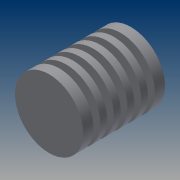
# Autodesk Inventor part: Ceramic_Spacer
Saved by Autodesk Inventor 2015 SP1 (Build 190203100, 203)
## iProperties
Created: 2015-09-10
Part Number: Ceramic_Spacer
Material: Generic
Document SubType Name: Modeling
Designer: nfitch
Density: 1 g/cm^3
Appearance: Default
Author: nfitch
Autodesk Inventor part; units mm, degrees
ref_plane "YZ Plane" through (0, 0, 0) normal (1, 0, 0) x (0, 1, 0)
ref_plane "XZ Plane" through (0, 0, 0) normal (0, 1, 0) x (-1, 0, 0)
ref_plane "XY Plane" through (0, 0, 0) normal (0, 0, 1) x (1, 0, 0)
sketch "Sketch1" plane through (0, 0, 0) normal (0, 1, 0) x (-1, 0, 0)
  circle A0 centre (0, 0) radius 5
  dimension "d0" = 10
  constraints: 1 centre point, 1 coincident
  measures "d0" diameter of A0
extrude "Extrusion1" add sketch "Sketch1" along normal blind 12
sketch "Sketch2" plane through (0, 0, 0) normal (1, 0, 0) x (0, 1, 0)
  line L0 (1.5, -2.5) -> (2.5, -2.5)
  line L1 (2.5, -2.5) -> (2.5, -7.5)
  line L2 (2.5, -7.5) -> (1.5, -7.5)
  line L3 (1.5, -7.5) -> (1.5, -2.5)
  line L4 (0, -5) -> (12, -5) projected
  line L5 (1.5, -2.5) -> (2.5, -7.5) construction
  line L6 (2.5, -2.5) -> (1.5, -7.5) construction
  line L7 (0, 0) -> (12, 0)
  line L8 (12, -5) -> (12, 5) projected
  line L9 (0, -10) -> (0, 7.5) projected
  line L10 (-2.4, 0) -> (14.4, 0) projected
  point P0 (2, -5)
  dimension "d3" = 1
  dimension "d4" = 5
  dimension "d9" = 2
  constraints: 14 end point, 3 midpoint, 2 parallel, 1 horizontal, 1 perpendicular, 1 point on line
  measures "d3" distance of L1.end L2.end
  measures "d4" distance of L0.end L1.end
  measures "d9" distance from line of L9 point (2, -5)
revolve "Revolution1" cut sketch "Sketch2" angle 360 about axis through (0, 0, 0) along (0, 1, 0) contours L0 L1 L4 L3 | L4 L1 L2 L3
pattern_linear "Rectangular Pattern1" count 5 spacing 2 along (0, 1, 0) of "Revolution1"
body "Solid1"
